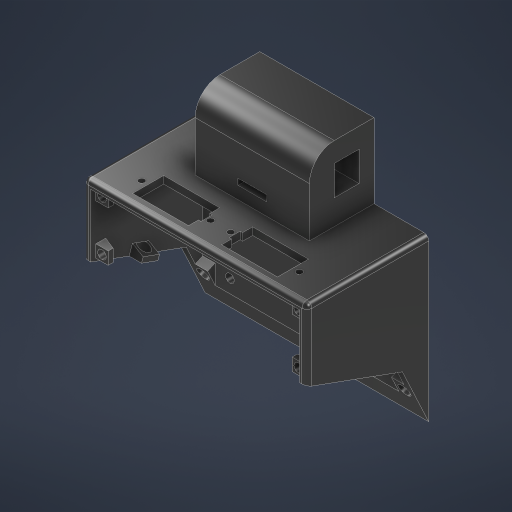
# Autodesk Inventor part: obudowa_robota
Saved by Autodesk Inventor 2023.4 (Build 274418000, 418)
## iProperties
Created: 2025-10-31
Part Number: obudowa_robota
Material: Tworzywo sztuczne PET
Document SubType Name: Modeling
Designer: Jakub Borsukiewicz
Density: 1.541 g/cm^3
Appearance: Lśniąca — czarna
Author: Jakub Borsukiewicz
Autodesk Inventor part; units mm, degrees
ref_plane "YZ Plane" through (0, 0, 0) normal (1, 0, 0) x (0, 1, 0)
ref_plane "XZ Plane" through (0, 0, 0) normal (0, 1, 0) x (-1, 0, 0)
sketch "Szkic1" plane through (0, 0, 0) normal (0, 0, 1) x (1, 0, 0)
  line L0 (-9, 0) -> (54, 0) projected
  line L1 (0, -19) -> (0, 114) projected
  line L2 (0, 0) -> (45, 0)
  line L3 (45, 0) -> (45, 65)
  line L4 (45, 65) -> (0, 65)
  line L5 (0, 65) -> (0, 0)
  line L6 (0, 65) -> (23, 65)
  line L7 (23, 65) -> (23, 95)
  line L8 (23, 95) -> (0, 95)
  line L9 (0, 95) -> (0, 65)
  point P0 (0, 95)
  dimension "d0" = 45
  dimension "d1" = 23
  dimension "d2" = 30
  dimension "d4" = 65
  constraints: 16 end point, 4 parallel, 2 horizontal, 2 perpendicular
  measures "d0" distance between parallel lines of L3 L1
  measures "d1" distance between parallel lines of L7 L9
  measures "d2" distance between parallel lines of L4 L8
  measures "d4" distance of L2.end L3.end
extrude "Wyciągnięcie proste1" add sketch "Szkic1" along normal blind 4
sketch "Szkic2" plane through (0, 0, 4) normal (0, 0, 1) x (1, 0, 0)
  line L0 (0, 95) -> (0, 0) projected
  line L1 (0, 0) -> (45, 0) projected
  line L2 (45, 0) -> (45, 65) projected
  line L3 (45, 65) -> (23, 65) projected
  line L4 (23, 65) -> (23, 95) projected
  line L5 (23, 95) -> (0, 95) projected
  line L6 (0, 0) -> (45, 0) projected
  line L7 (42, 0) -> (42, 62)
  line L8 (45, 65) -> (23, 65) projected
  line L9 (45, 0) -> (45, 65) projected
  line L10 (42, 62) -> (8, 62)
  line L11 (23, 95) -> (0, 95) projected
  line L12 (8, 62) -> (8, 92)
  line L13 (8, 92) -> (0, 92)
  dimension "d7" = 3
  dimension "d9" = 3
  dimension "d13" = 15
  dimension "d14" = 3
  constraints: 8 end point, 2 perpendicular, 2 point on line, 1 horizontal, 1 vertical
  measures "d7" distance between parallel lines of L2 L7
  measures "d9" distance between parallel lines of L3 L10
  measures "d13" distance between parallel lines of L4 L12
  measures "d14" distance between parallel lines of L5 L13
extrude "Wyciągnięcie proste2" add sketch "Szkic2" along normal blind 45 contours L5 L4 L3 L2 L1 L7 L10 L12 L13 L0
sketch "Szkic3" plane through (23, 65, 0) normal (1, 0, 0) x (0, 0, -1)
  line L0 (0, 0) -> (0, 30) projected
  line L1 (0, 30) -> (-49, 30) projected
  line L2 (-49, 0) -> (-49, 30) projected
  line L3 (0, 0) -> (-49, 0) projected
  line L4 (-16, 10) -> (-6, 10)
  line L5 (-6, 10) -> (-6, 22)
  line L6 (-6, 22) -> (-16, 22)
  line L7 (-16, 22) -> (-16, 10)
  point P0 (0, -65)
  point P1 (-16, 16)
  point P2 (-11, 22)
  dimension "d15" = 10
  dimension "d16" = 12
  dimension "d18" = 14
  dimension "d19" = 11
  constraints: 8 end point, 2 midpoint, 2 parallel, 1 horizontal, 1 perpendicular
  measures "d15" distance of L6.end L5.end
  measures "d16" distance of L6.end L4.start
  measures "d18" distance from line of L1 point (-16, 16)
  measures "d19" distance from line of L0 point (-11, 22)
extrude "Wyciągnięcie proste3" cut sketch "Szkic3" against normal blind 50 contours L7 L6 L5 L4
sketch "Szkic4" plane through (0, 0, 49) normal (0, 0, 1) x (1, 0, 0)
  line L0 (23, 95) -> (0, 95) projected
  line L1 (0, 95) -> (0, 92) projected
  line L2 (0, 92) -> (8, 92) projected
  line L3 (8, 92) -> (8, 62) projected
  line L4 (8, 62) -> (42, 62) projected
  line L5 (42, 62) -> (42, 0) projected
  line L6 (42, 0) -> (45, 0) projected
  line L7 (45, 0) -> (45, 65) projected
  line L8 (45, 65) -> (23, 65) projected
  line L9 (23, 65) -> (23, 95) projected
  line L10 (45, 65) -> (23, 65) projected
  line L11 (23, 65) -> (8, 65)
  line L12 (8, 92) -> (8, 62) projected
  point P0 (0, 0)
  constraints: 2 end point, 1 perpendicular, 1 point on line
extrude "Wyciągnięcie proste4" cut sketch "Szkic4" against normal blind 23 contours L9 L11 L3 L2 L1 L0
sketch "Szkic7" plane through (23, 65, 0) normal (1, 0, 0) x (0, 0, -1)
  line L0 (-26, 30) -> (-26, 0) projected
  line L1 (0, 0) -> (-26, 0) projected
  line L2 (0, 0) -> (0, 30) projected
  line L3 (0, 30) -> (-26, 30) projected
  line L4 (-16, 22) -> (-6, 22) projected
  line L5 (-6, 22) -> (-6, 10) projected
  line L6 (-6, 10) -> (-16, 10) projected
  line L7 (-16, 10) -> (-16, 22) projected
  circle A0 centre (-11, 16) radius 14
  point P0 (0, -65)
  dimension "d33" = 28
  constraints: 1 centre point
  measures "d33" diameter of A0
sketch "Szkic8" plane through (8, 62, 4) normal (-1, 0, 0) x (0, 0, 1)
  line L0 (45, 3) -> (22, 3) projected
  line L1 (22, 3) -> (22, 30) projected
  line L2 (0, 30) -> (22, 30) projected
  line L3 (0, 0) -> (0, 30) projected
  line L4 (0, 0) -> (45, 0) projected
  line L5 (45, 3) -> (45, 0) projected
  line L6 (2, 25) -> (12, 25) projected
  line L7 (12, 25) -> (12, 13) projected
  line L8 (12, 13) -> (2, 13) projected
  line L9 (2, 13) -> (2, 25) projected
  line L10 (0, 30) -> (22, 30) projected
  line L11 (19, 30) -> (19, 0)
  line L12 (0, 0) -> (45, 0) projected
  point P0 (-4, -62)
  dimension "d34" = 3
  constraints: 2 end point, 2 point on line, 1 vertical
  measures "d34" distance between parallel lines of L11 L1
extrude "Wyciągnięcie proste6" add sketch "Szkic8" along normal up to surface (8 mm away) contours L5 L4 L11 L2 L1 L0
sketch "Szkic9" plane through (23, 65, 0) normal (0, 1, 0) x (1, 0, 0)
  line L0 (22, 0) -> (0, 0) projected
  line L1 (0, 0) -> (0, -26) projected
  line L2 (0, -26) -> (-23, -26) projected
  line L3 (-23, -26) -> (-23, -49) projected
  line L4 (22, -49) -> (-23, -49) projected
  line L5 (22, 0) -> (22, -49) projected
  line L6 (10.8, -45) -> (-21, -45)
  line L7 (-21, -45) -> (-21, -32.5)
  line L8 (-21, -32.5) -> (10.8, -32.5)
  line L9 (10.8, -32.5) -> (10.8, -45)
  line L10 (6.15, -45) -> (6.15, -32.5)
  line L11 (-16.35, -45) -> (-16.35, -32.5)
  circle A0 centre (-18.95, -38.75) radius 1.25
  circle A1 centre (8.75, -38.75) radius 1.25
  line L12 (-16.35, -41) -> (-17.35, -41)
  line L13 (-17.35, -41) -> (-17.35, -36.5)
  line L14 (-17.35, -36.5) -> (-16.35, -36.5)
  line L15 (-16.35, -36.5) -> (-16.35, -41)
  point P0 (-23, 0)
  point P1 (6.15, -41)
  dimension "d89" = 31.8
  dimension "d90" = 12.5
  dimension "d91" = 4.65
  dimension "d92" = 4.65
  dimension "d93" = 2.5
  dimension "d94" = 2.5
  dimension "d95" = 6.25
  dimension "d96" = 6.25
  dimension "d97" = 27.7
  dimension "d98" = 2.05
  dimension "d103" = 4
  dimension "d160" = 1
  dimension "d161" = 4
  dimension "d162" = 4
  dimension "d163" = 2
  constraints: 20 end point, 6 point on line, 4 parallel, 4 perpendicular, 2 centre point, 2 horizontal
  measures "d89" distance of L6.start L6.end
  measures "d90" distance of L6.end L7.end
  measures "d91" distance between parallel lines of L7 L11
  measures "d92" distance between parallel lines of L9 L10
  measures "d93" diameter of A1
  measures "d94" diameter of A0
  measures "d95" distance from line of L8 A0.centre
  measures "d96" distance from line of L8 A1.centre
  measures "d97" distance of A1.centre A0.centre
  measures "d98" distance from line of L9 A1.centre
  measures "d103" distance between parallel lines of L4 L6
  measures "d160" distance of L13.end L14.end
  measures "d161" distance between parallel lines of L8 L14
  measures "d162" distance between parallel lines of L12 L6
  measures "d163" distance between parallel lines of L3 L7
extrude "Wyciągnięcie proste7" cut sketch "Szkic9" against normal blind 15 contours L6 L11 L8 L10 | L12 L13 L14 L11 | A0 | A1
sketch "Szkic10" plane through (0, 0, 4) normal (0, 0, 1) x (1, 0, 0)
  line L0 (42, 0) -> (42, 62) projected
  line L1 (42, 62) -> (8, 62) projected
  line L2 (8, 62) -> (8, 92) projected
  line L3 (8, 92) -> (0, 92) projected
  line L4 (0, 92) -> (0, 0) projected
  line L5 (0, 0) -> (42, 0) projected
  line L6 (35, 12) -> (27, 12)
  line L7 (27, 12) -> (27, 25)
  line L8 (27, 25) -> (35, 25)
  line L9 (35, 25) -> (35, 12)
  line L10 (34.5, 18) -> (27.5, 18)
  line L11 (27.5, 18) -> (27.5, 24)
  line L12 (27.5, 24) -> (34.5, 24)
  line L13 (34.5, 24) -> (34.5, 18)
  circle A0 centre (31, 14) radius 1.75
  dimension "d52" = 13
  dimension "d53" = 8
  dimension "d54" = 6
  dimension "d55" = 7
  dimension "d56" = 0.5
  dimension "d57" = 1
  dimension "d58" = 4
  dimension "d59" = 3.5
  dimension "d60" = 2
  dimension "d61" = 7
  dimension "d62" = 12
  constraints: 16 end point, 4 parallel, 2 horizontal, 2 perpendicular, 1 centre point
  measures "d52" distance of L6.end L7.end
  measures "d53" distance of L7.end L8.end
  measures "d54" distance of L10.end L11.end
  measures "d55" distance of L10.start L10.end
  measures "d56" distance between parallel lines of L7 L11
  measures "d57" distance between parallel lines of L8 L12
  measures "d58" distance from line of L7 A0.centre
  measures "d59" diameter of A0
  measures "d60" distance from line of L6 A0.centre
  measures "d61" distance between parallel lines of L0 L9
  measures "d62" distance between parallel lines of L5 L6
extrude "Wyciągnięcie proste8" cut sketch "Szkic10" against normal blind 15 contours L10 L11 L12 L13 | A0
sketch "Szkic11" plane through (45, 0, 0) normal (1, 0, 0) x (0, 0, -1)
  line L0 (0, 0) -> (-4, 0) projected
  line L1 (-49, 0) -> (-49, 65) projected
  line L2 (-49, 65) -> (-49, 36.6467)
  line L3 (0, 0) -> (0, 65) projected
  line L4 (-49, 0) -> (-49, 65) projected
  line L5 (0, 0) -> (-49, 0) projected
  line L6 (0, 0) -> (-10.5655, 22.6577)
  line L7 (-10.5655, 22.6577) -> (-49, 36.6467)
  line L8 (0, 65) -> (-49, 65) projected
  point P0 (0, 0)
  dimension "d66" = 25
  dimension "d67" = 25
  dimension "d104" = 135
  constraints: 6 end point, 1 point on line
  measures "d66" distance of L3.start L6.end
  measures "d67" angle of L3 L6
  measures "d104" angle of L6 L7
extrude "Wyciągnięcie proste9" cut sketch "Szkic11" against normal blind 50 contours L0 L5 L1 L7 L6
sketch "Szkic13" plane through (0, 0, 4) normal (0, 0, 1) x (1, 0, 0)
  line L0 (0, 8.578) -> (42, 8.578) projected
  line L1 (42, 8.578) -> (42, 62) projected
  line L2 (42, 62) -> (8, 62) projected
  line L3 (8, 62) -> (8, 92) projected
  line L4 (8, 92) -> (0, 92) projected
  line L5 (0, 92) -> (0, 8.578) projected
  circle A0 centre (31, 14) radius 1.75 projected
  line L6 (27.5, 18) -> (27.5, 24) projected
  line L7 (27.5, 24) -> (34.5, 24) projected
  line L8 (34.5, 24) -> (34.5, 18) projected
  line L9 (34.5, 18) -> (27.5, 18) projected
  circle A1 centre (34, 44) radius 1.75
  line L10 (0, 92) -> (0, 8.578) projected
  point P0 (0, 0)
  dimension "d72" = 3.5
  dimension "d150" = 18
  dimension "d151" = 8
  constraints: 1 centre point
  measures "d72" diameter of A1
  measures "d150" distance from line of L2 A1.centre
  measures "d151" distance from line of L1 A1.centre
extrude "Wyciągnięcie proste10" cut sketch "Szkic13" against normal blind 3 contours A1
fillet "Zaokrąglenie1" radius 2 1 edges at (45, 65, 24.5)
fillet "Zaokrąglenie2" radius 2 3 edges at (21.5, 65, 49) (44.4142, 64.4142, 49) (45, 49.8234, 49)
fillet "Zaokrąglenie3" radius 7 1 edges at (4, 92, 23)
fillet "Zaokrąglenie5" radius 5 1 edges at (4, 92, 4)
fillet "Zaokrąglenie4" radius 10 1 edges at (11.5, 95, 26)
sketch "Szkic19" plane through (0, 0, 0) normal (0, -0.4226183, 0.9063078) x (1, 0, 0)
  line L0 (0, 0) -> (0, 9.4648) projected
  line L1 (0, 0) -> (45, 0) projected
  line L2 (45, 25) -> (45, 0) projected
  line L3 (45, 25) -> (42, 25) projected
  line L4 (42, 9.4648) -> (42, 25) projected
  line L5 (0, 9.4648) -> (42, 9.4648) projected
  line L6 (42, 9.4648) -> (42, 57.8816) projected
  line L7 (42, 9.4648) -> (37, 9.4648)
  line L8 (37, 9.4648) -> (37, 16.4648)
  line L9 (37, 16.4648) -> (42, 16.4648)
  line L10 (42, 16.4648) -> (42, 9.4648)
  dimension "d107" = 5
  dimension "d108" = 7
  constraints: 8 end point, 2 parallel, 1 horizontal, 1 perpendicular
  measures "d107" distance of L8.end L9.end
  measures "d108" distance of L7.end L8.end
extrude "Wyciągnięcie proste15" add sketch "Szkic19" against normal blind 4 contours L8 L9 L4 L5
sketch "Szkic20" plane through (0, 0, 0) normal (0, -0.4226183, 0.9063078) x (1, 0, 0)
  line L0 (0, 0) -> (0, 9.4648) projected
  line L1 (0, 0) -> (45, 0) projected
  line L2 (45, 25) -> (45, 0) projected
  line L3 (45, 25) -> (42, 25) projected
  line L4 (42, 16.4648) -> (42, 25) projected
  line L5 (42, 16.4648) -> (37, 16.4648) projected
  line L6 (37, 16.4648) -> (37, 9.4648) projected
  line L7 (0, 9.4648) -> (37, 9.4648) projected
  point P0 (40.5, 12.4648)
  dimension "d111" = 3.5
  dimension "d112" = 4
  measures "d111" distance from line of L6 point (40.5, 12.465)
  measures "d112" distance from line of L5 point (40.5, 12.465)
hole "Otwór1" at (40.5, 11.297, 5.2679) direction (0, 0.4226183, -0.9063078) diameter 5 depth 4
sketch "Szkic22" plane through (42, 22.6577, 10.5655) normal (0, -0.9396926, 0.3420201) x (1, 0, 0)
  ellipse E0 centre (1, 38.7728) end of major axis (1, 40.9012) minor radius 2 (3, 38.7728) -> (1, 40.9012) ccw projected
  line L0 (0, 40.9012) -> (1, 40.9012) projected
  line L1 (0, 0) -> (0, 40.9012) projected
  line L2 (3, 0) -> (0, 0) projected
  line L3 (3, 38.7728) -> (3, 0) projected
  line L4 (0, 0) -> (0, 40.9012) projected
  line L5 (0, 17.5) -> (-5, 17.5)
  line L6 (-5, 17.5) -> (-5, 24.5)
  line L7 (-5, 24.5) -> (0, 24.5)
  line L8 (0, 24.5) -> (0, 17.5)
  point P0 (-42, -17.6777)
  point P1 (0, 17.5)
  point P2 (0, 24.5)
  dimension "d120" = 5
  dimension "d121" = 7
  dimension "d122" = 17.5
  constraints: 8 end point, 2 parallel, 1 horizontal, 1 perpendicular, 1 point on line, 1 other
  measures "d120" distance of L6.end L7.end
  measures "d121" distance of L5.end L6.end
  measures "d122" distance between parallel lines of L2 L5
extrude "Wyciągnięcie proste16" add sketch "Szkic22" against normal blind 4 contours L1 L5 L6 L7
sketch "Szkic23" plane through (42, 22.6577, 10.5655) normal (0, -0.9396926, 0.3420201) x (1, 0, 0)
  ellipse E0 centre (1, 38.7728) end of major axis (1, 40.9012) minor radius 2 (3, 38.7728) -> (1, 40.9012) ccw projected
  line L0 (0, 40.9012) -> (1, 40.9012) projected
  line L1 (0, 24.5) -> (0, 40.9012) projected
  line L2 (0, 24.5) -> (-5, 24.5) projected
  line L3 (-5, 24.5) -> (-5, 17.5) projected
  line L4 (-5, 17.5) -> (0, 17.5) projected
  line L5 (0, 0) -> (0, 17.5) projected
  line L6 (3, 0) -> (0, 0) projected
  line L7 (3, 38.7728) -> (3, 0) projected
  point P0 (-42, -17.6777)
  point P1 (-1.5, 21)
  dimension "d125" = 3.5
  dimension "d126" = 3.5
  constraints: 1 other
  measures "d125" distance from line of L2 point (-1.5, 21)
  measures "d126" distance from line of L3 point (-1.5, 21)
hole "Otwór2" at (40.5, 29.8401, 30.299) direction (0, 0.9396926, -0.3420201) diameter 5 depth 4
sketch "Szkic27" plane through (0, 0, 26) normal (0, 0, 1) x (1, 0, 0)
  line L0 (0, 85) -> (23, 85) projected
  line L1 (0, 85) -> (0, 65) projected
  line L2 (23, 65) -> (0, 65) projected
  line L3 (23, 85) -> (23, 65) projected
  line L4 (0, 70) -> (5.75, 70)
  line L5 (5.75, 70) -> (5.75, 72.5)
  line L6 (5.75, 72.5) -> (0, 72.5)
  line L7 (0, 72.5) -> (0, 70)
  point P0 (0, 0)
  point P1 (0, 72.5)
  dimension "d155" = 5.75
  dimension "d156" = 2.5
  dimension "d157" = 5
  constraints: 8 end point, 2 parallel, 1 horizontal, 1 perpendicular, 1 point on line
  measures "d155" distance of L6.end L5.end
  measures "d156" distance of L4.end L5.end
  measures "d157" distance between parallel lines of L4 L2
extrude "Wyciągnięcie proste18" cut sketch "Szkic27" against normal blind 10 contours L6 L5 L4 L1
ref_plane "Płaszczyzna konstrukcyjna1" through (0, 0, 47) normal (0, 0, 1) x (1, 0, 0)
sketch "Szkic30" plane through (0, 0, 47) normal (0, 0, 1) x (1, 0, 0)
  line L0 (37, 16.3017) -> (42, 16.3017) projected
  line L1 (42, 16.3017) -> (42, 62) projected
  line L2 (42, 62) -> (8, 62) projected
  line L3 (8, 62) -> (8, 87) projected
  line L4 (0, 87) -> (8, 87) projected
  line L5 (0, 87) -> (0, 8.578) projected
  line L6 (0, 8.578) -> (37, 8.578) projected
  line L7 (37, 8.578) -> (37, 16.3017) projected
  line L8 (27.5, 18) -> (27.5, 24) projected
  line L9 (27.5, 24) -> (34.5, 24) projected
  line L10 (34.5, 24) -> (34.5, 18) projected
  line L11 (34.5, 18) -> (27.5, 18) projected
  circle A0 centre (31, 14) radius 1.75 projected
  circle A1 centre (34, 44) radius 1.75 projected
  line L12 (42, 62) -> (8, 62) projected
  line L13 (42, 62) -> (37, 62)
  line L14 (37, 62) -> (37, 57)
  line L15 (37, 57) -> (42, 57)
  line L16 (42, 57) -> (42, 62)
  ellipse E0 centre (40.5, 29.8401) end of major axis (43, 29.8401) minor radius 0.8551 projected
  ellipse E1 centre (43, 35.9188) end of major axis (45, 35.9188) minor radius 0.7279 (45, 35.9188) -> (43, 36.6467) ccw projected
  line L17 (42, 36.6467) -> (43, 36.6467) projected
  line L18 (42, 31.0372) -> (42, 36.6467) projected
  line L19 (42, 31.0372) -> (37, 31.0372) projected
  line L20 (37, 31.0372) -> (37, 28.643) projected
  line L21 (37, 28.643) -> (42, 28.643) projected
  line L22 (42, 22.6577) -> (42, 28.643) projected
  line L23 (45, 22.6577) -> (42, 22.6577) projected
  line L24 (45, 35.9188) -> (45, 22.6577) projected
  line L25 (42, 37) -> (37, 37)
  line L26 (37, 37) -> (37, 42)
  line L27 (37, 42) -> (42, 42)
  line L28 (42, 42) -> (42, 37)
  circle A2 centre (39.5, 39.5) radius 1.75
  circle A3 centre (39.5, 59.5) radius 1.75
  point P0 (0, 0)
  point P1 (37, 39.5)
  point P2 (39.5, 37)
  dimension "d173" = 5
  dimension "d174" = 5
  dimension "d175" = 5
  dimension "d176" = 5
  dimension "d177" = 3.5
  dimension "d178" = 3.5
  dimension "d179" = 2.5
  dimension "d180" = 2.5
  dimension "d181" = 2.5
  dimension "d182" = 2.5
  dimension "d183" = 20
  constraints: 16 end point, 4 parallel, 2 centre point, 2 horizontal, 2 midpoint, 2 perpendicular, 1 point on line, 1 other
  measures "d173" distance of L15.end L14.end
  measures "d174" distance of L13.end L14.end
  measures "d175" distance of L26.end L27.end
  measures "d176" distance of L25.end L26.end
  measures "d177" diameter of A2
  measures "d178" diameter of A3
  measures "d179" distance from line of L14 A3.centre
  measures "d180" distance from line of L15 A3.centre
  measures "d181" distance of point (37, 39.5) A2.centre
  measures "d182" distance of point (39.5, 37) A2.centre
  measures "d183" distance of A3.centre A2.centre
extrude "Wyciągnięcie proste19" add sketch "Szkic30" against normal blind 4 contours L2 L1 L15 L14 | L25 L26 L27 L1
chamfer "Faza2" distance 5 distance2 2 1 edges at (37, 59.5, 43)
chamfer "Faza3" distance 5 distance2 2 1 edges at (37, 39.5, 43)
chamfer "Faza4" distance 5 distance2 2 1 edges at (37, 33.5989, 28.9309)
mirror "Odbij5" about plane through (0, 0, 0) normal (1, 0, 0) of "Wyciągnięcie proste1", "Wyciągnięcie proste2", "Wyciągnięcie proste3", "Wyciągnięcie proste4", "Wyciągnięcie proste6", "Wyciągnięcie proste7", "Wyciągnięcie proste8", "Wyciągnięcie proste9", "Wyciągnięcie proste10", "Zaokrąglenie1", "Zaokrąglenie2", "Zaokrąglenie3", "Zaokrąglenie5", "Zaokrąglenie4", "Wyciągnięcie proste15", "Otwór1", "Wyciągnięcie proste16", "Otwór2", "Wyciągnięcie proste18", "Wyciągnięcie proste19", "Faza2", "Faza3", "Faza4"
sketch "Szkic31" plane through (-23, 65, 0) normal (-1, 0, 0) x (0, 0, 1)
  line L0 (6, 22) -> (16, 22) projected
  line L1 (16, 22) -> (16, 10) projected
  line L2 (16, 10) -> (6, 10) projected
  line L3 (6, 10) -> (6, 22) projected
  arc A0 (26, 20) -> (16, 30) centre (16, 20) ccw projected
  line L4 (0, 30) -> (16, 30) projected
  line L5 (0, 0) -> (0, 30) projected
  line L6 (0, 0) -> (26, 0) projected
  line L7 (26, 0) -> (26, 20) projected
  circle A1 centre (11, 16) radius 14
  point P0 (0, -65)
  dimension "d195" = 28
  constraints: 1 centre point
  measures "d195" diameter of A1
